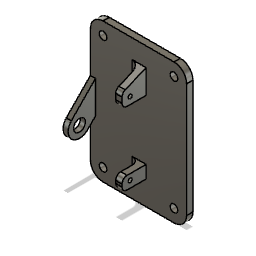
mota_ita v4 (Autodesk Fusion 360 design; units mm, degrees)
Autodesk Fusion 360 part; units mm, degrees
note: some values were not read from the file. Chosen so that the rebuilt part matches the saved one: which bodies a step acts on. Set by a fixed rule: which sketch regions a step uses.
sketch "スケッチ2" plane through (0, 0, 0) normal (0, 0, 1) x (1, 0, 0)
  line L0 (-17, 34) -> (17, 34)
  line L1 (-17, -21.05) -> (-17, 34)
  line L2 (17, 34) -> (17, -21.05)
  line L3 (17, -21.05) -> (-17, -21.05)
  line L4 (0, 39) -> (0, -27)
  line L5 (-28, 0) -> (24, 0)
  line L6 (-14, 34) -> (14, 34)
  line L7 (19, 29) -> (19, -16.05)
  line L8 (14, -21.05) -> (-14, -21.05)
  line L9 (-19, -16.05) -> (-19, 29)
  line L10 (-19, -11.05) -> (-19, 0)
  line L11 (19, 0) -> (19, -11.05)
  arc A0 (-14, 34) -> (-19, 29) centre (-14, 29) ccw
  arc A1 (19, 29) -> (14, 34) centre (14, 29) ccw
  arc A2 (-19, -16.05) -> (-14, -21.05) centre (-14, -16.05) ccw
  arc A3 (14, -21.05) -> (19, -16.05) centre (14, -16.05) ccw
  circle A4 centre (-14, 29) radius 1.5
  circle A5 centre (14, 29) radius 1.5
  circle A6 centre (-14, -16.05) radius 1.5
  circle A7 centre (14, -16.05) radius 1.5
  dimension "d40" = 34
  dimension "d44" = 34
  dimension "d45" = 2
  dimension "d46" = 2
  dimension "d49" = 5
  dimension "d127" = 21.05
  dimension "d130" = 5
  dimension "d131" = 5
  dimension "d132" = 3
  dimension "d133" = 3
  dimension "d134" = 3
  dimension "d135" = 3
  constraint horizontal L0
  constraint vertical L2
  constraint horizontal L3
  constraint vertical L1
  constraint perpendicular L3 L4
  constraint perpendicular L1 L5
  constraint coincident origin L4
  constraint coincident origin L5
  constraint symmetric L1 L2 L4
  constraint horizontal L6
  constraint vertical L7
  constraint horizontal L8
  constraint vertical L9
  constraint collinear L0 L6
  constraint collinear L3 L8
  constraint vertical L10
  constraint vertical L11
  constraint collinear L7 L11
  constraint collinear L9 L10
  constraint tangent L6 A0
  constraint tangent L9 A0
  constraint tangent L6 A1
  constraint tangent L7 A1
  constraint equal A0 A1
  constraint tangent L8 A2
  constraint tangent L9 A2
  constraint tangent L7 A3
  constraint tangent L8 A3
  constraint concentric A0 A4
  constraint concentric A1 A5
  constraint concentric A2 A6
  constraint concentric A3 A7
  measures "d40" distance of L1 L2
  measures "d44" distance of origin L0
  measures "d45" distance of L1 L9
  measures "d46" distance of L2 L7
  measures "d49" radius of A0
  measures "d127" distance of origin L8
  measures "d130" radius of A2
  measures "d131" radius of A3
  measures "d132" diameter of A4
  measures "d133" diameter of A5
  measures "d134" diameter of A6
  measures "d135" diameter of A7
extrude "押し出し1" add sketch "スケッチ2" against normal blind 2.5 contours L0 L1 L4 L5 L6 A0 | L1 L5 L9 A0 | L0 L2 L4 L5 L6 A1 | L1 L3 L4 L5 L8 A2 | L1 L5 L9 L10 A2 | L2 L3 L4 L5 L8 A3 | L2 L5 L7 A1 | L2 L5 L7 L11 A3 makes body 1
sketch "スケッチ1" plane through (0, 0, 0) normal (1, 0, 0) x (0, 0, -1)
  line L0 (0, 48.5158) -> (0, -21.5258)
  line L1 (-30.4996, 0) -> (69.8846, 0)
  line L2 (0, 26.05) -> (0, 16.55)
  line L3 (0, 16.55) -> (-7.5, 16.55)
  line L4 (0, -6.05) -> (-7.5, -6.05)
  line L5 (-9.5, -8.05) -> (-9.5, -9.05)
  line L6 (-7.5, -11.05) -> (0, -11.05)
  line L7 (0, -11.05) -> (0, -6.05)
  circle A0 centre (-6.3, -8.3) radius 0.8
  circle A1 centre (-6.3, 19.3) radius 0.8
  line L8 (0, 34) -> (0, -21.05)
  line L9 (-9.5, 18.55) -> (-9.5, 20.722)
  line L10 (-8.2761, 22.5653) -> (0, 26.05)
  circle A2 centre (-6.3, 0) radius 2.35
  circle A3 centre (-6.3, 0) radius 4.5
  line L11 (-9.5143, 3.1493) -> (0, 12.8598)
  line L12 (-3.0857, -3.1493) -> (0, 0)
  arc A4 (-8.2761, 22.5653) -> (-9.5, 20.722) centre (-7.5, 20.722) ccw
  arc A5 (-9.5, 18.55) -> (-7.5, 16.55) centre (-7.5, 18.55) ccw
  arc A6 (-7.5, -6.05) -> (-9.5, -8.05) centre (-7.5, -8.05) ccw
  arc A7 (-9.5, -9.05) -> (-7.5, -11.05) centre (-7.5, -9.05) ccw
  point P0 (-9.5, 16.55)
  point P1 (-9.5, 22.05)
  dimension "d5" = 5
  dimension "d20" = 1.6
  dimension "d21" = 1.6
  dimension "d22" = 27.6
  dimension "d23" = 8.3
  dimension "d24" = 6.3
  dimension "d25" = 6.3
  dimension "d26" = 9.5
  dimension "d27" = 2.75
  dimension "d28" = 5.5
  dimension "d30" = 6.3
  dimension "d31" = 4.7
  dimension "d32" = 9
  dimension "d34" = 2
  dimension "d35" = 2
  dimension "d70" = 2.75
  dimension "d126" = 26.05
  constraint vertical L0
  constraint horizontal L1
  constraint coincident L12.end L0
  constraint coincident L12.end L1
  constraint vertical L2
  constraint horizontal L3
  constraint horizontal L4
  constraint vertical L5
  constraint horizontal L6
  constraint vertical L7
  constraint collinear L0 L2
  constraint collinear L0 L7
  constraint perpendicular L3 L9
  constraint collinear L5 L9
  constraint coincident L1 A2.centre
  constraint concentric A2 A3
  constraint coincident A3 L11.start
  constraint tangent A3 L11
  constraint coincident L0 L11.end
  constraint coincident A3 L12.start
  constraint tangent A3 L12
  constraint coincident L8 L12.end
  constraint parallel L11 L12
  constraint coincident L12.end origin
  constraint coincident P1 L9
  constraint coincident P1 L10
  constraint tangent L9 A4
  constraint tangent L10 A4
  constraint coincident P0 L3
  constraint coincident P0 L9
  constraint tangent L3 A5
  constraint tangent L9 A5
  constraint equal A4 A5
  constraint tangent L4 A6
  constraint tangent L5 A6
  constraint tangent L5 A7
  constraint tangent L6 A7
  constraint equal A6 A7
  measures "d5" distance of L4 L6
  measures "d20" diameter of A0
  measures "d21" diameter of A1
  measures "d22" vertical distance of A0.centre A1.centre
  measures "d23" vertical distance of A0.centre L12.end
  measures "d24" distance of A0.centre L8
  measures "d25" horizontal distance of A1.centre L12.end
  measures "d26" distance of L5 L8
  measures "d27" distance of L3 A1.centre
  measures "d28" distance of P0 P1
  measures "d30" distance of L12.end A2.centre
  measures "d31" diameter of A2
  measures "d32" diameter of A3
  measures "d34" radius of A4
  measures "d35" radius of A6
  measures "d70" distance of L6 A0.centre
  measures "d126" distance of L12.end L2.start
extrude "押し出し2" add sketch "スケッチ1" along normal blind 3 separate body contours L0 L2 L3 L8 L9 L10 A4 A5 | L0 L4 L5 L6 L7 L8 A6 A7 makes body 2 at (0, 20.7119, 1.8452) makes body 3 at (0, -8.4667, 1.8333)
extrude "押し出し3" cut sketch "スケッチ1" along normal blind 0.5 contours L0 L2 L3 L8 L9 L10 A4 A5 | L0 L4 L5 L6 L7 L8 A6 A7 bodies 1 2 3
extrude "押し出し4" add sketch "スケッチ1" against normal blind 19 contours L0 L1 L8 A3 L11 | L1 A3 L12 | L1 A2 A3 | L1 A2 A3 bodies 3 makes body 4
extrude "押し出し5" cut sketch "スケッチ1" against normal blind 17 contours L0 L1 L8 A3 L11 | L1 A3 L12 | L1 A2 A3 | L1 A2 A3 bodies 1 2 3 4
combine "結合1" operation add target body 1 tool bodies 3 2 4
fillet "フィレット3" radius 3 1 edges at (0.5, -8.55, 0) on bodies 1
fillet "フィレット4" radius 3 1 edges at (0.5, 21.3, 0) on bodies 1
split "分割1" by plane through (0, 0, 0) normal (0, 0, 1) bodies 1 makes body 5 at (3, -8.4667, 1.8333) makes body 6 at (-19, 4.8194, 1.5258) makes body 7 at (3, 20.7119, 1.8452)
move_body "移動1" bodies 7 to x (1, 0, 0) y (0, 1, 0) z (0, 0, 1) at (0, 0.5, 0)
move_body "移動2" bodies 5 to x (1, 0, 0) y (0, 1, 0) z (0, 0, 1) at (0, -0.5, 0)
combine "結合2" operation add target body 5 tool bodies 1 6 7
copy_body "ボディ -> コンポーネント5" bodies 5 removing the originals makes body 8 in component "Component"
component "Component" placed x (1, 0, 0) y (0, 1, 0) z (0, 0, 1) at (0, 0, 0)
